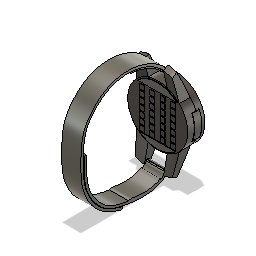
self-sus-wearable (Autodesk Fusion 360 design; units mm, degrees)
part number: Configuration 2
Autodesk Fusion 360 part; units mm, degrees
note: some values were not read from the file. Set by a fixed rule: which face or edge a step refers to.
(part 1 of 2)
sketch "Sketch1" plane through (0, 0, 0) normal (0, 1, 0) x (1, 0, 0)
  line L0 (0, 0) -> (0, 36)
  line L1 (0, 36) -> (-13.5946, 42.3393)
  line L2 (-13.5946, 42.3393) -> (-13.5946, 41.2357)
  line L3 (-13.5946, 41.2357) -> (-13.5946, 31.2357)
  line L4 (-13.5946, 31.2357) -> (-17.5946, 31.2357)
  line L5 (-17.5946, 31.2357) -> (-17.5946, 0)
  line L6 (-17.5946, 0) -> (0, 0)
  line L7 (-62.5946, 50) -> (-62.5946, 0)
  dimension "d1" = 36
  dimension "d2" = 15
  dimension "d5" = 65
  dimension "d6" = 10
  dimension "d7" = 4
  dimension "d11" = 45
  dimension "d12" = 31.2357
  constraint coincident L0.start L6.end
  constraint vertical L0
  constraint vertical L3
  constraint perpendicular L3 L4
  constraint perpendicular L4 L5
  constraint perpendicular L0 L6
  constraint vertical L7
  measures "d1" distance of L0.start L0.end
  measures "d2" distance of L0.end L1.end
  measures "d5" angle of L0 L1
  measures "d6" distance of L2.end L3.end
  measures "d7" distance of L3.end L4.end
  measures "d11" distance of L5 L7
  measures "d12" distance of L4.end L5.end
sketch "Sketch2" plane through (0, 0, 0) normal (0, 1, 0) x (1, 0, 0)
  line L0 (-62.5946, 45) -> (-62.5946, 0)
  line L1 (-17.5946, 31.2357) -> (-17.5946, 0)
  line L2 (0, 36) -> (-13.5946, 42.3393)
  dimension "d8" = 45
  constraint vertical L0
  measures "d8" distance of L0 L1
revolve "Revolve1" add sketch "Sketch1" angle 360 about axis through (-62.5946, 0, -45) along (0, 0, 1) makes body 1
sketch "Sketch3" plane through (0, 0, 0) normal (1, 0, 0) x (0, 0, -1)
  line L0 (20, 0) -> (7.7499, 0)
  line L1 (20, 0) -> (21.7425, 0)
  constraint horizontal L0
sketch "Sketch4" plane through (0, 0, 0) normal (0, 1, 0) x (1, 0, 0)
  line L0 (0.0672, 22.9643) -> (40, 1.7316)
  line L1 (40, 1.7316) -> (34.8066, -8.0357)
  line L2 (34.8066, -8.0357) -> (0, 0)
  line L3 (1.75, 0) -> (22.5, 0)
  line L4 (0, 20) -> (0, 7.7499)
  line L5 (0.0672, 22.9643) -> (0, 0)
  dimension "d14" = 13
  dimension "d15" = 28
  dimension "d16" = 40
  dimension "d17" = 31
  constraint perpendicular L0 L1
  constraint coincident L2.end L5.end
  measures "d14" angle of L2 L3
  measures "d15" angle of L0 L3
  measures "d16" distance of L0.end L4
  measures "d17" vertical distance of L0.start L1.end
revolve "Revolve2" add sketch "Sketch4" angle 360 about axis through (-62.5946, 0, 0) along (0, 0, -1) bodies 1
sketch "Sketch5" plane through (0, 0, 0) normal (0, 1, 0) x (1, 0, 0)
  line L0 (-40, 0) -> (-50, 0)
  constraint horizontal L0
sketch "Sketch6" plane through (0, 0, 0) normal (0, 0, 1) x (1, 0, 0)
  line L0 (-42.5946, 123.9624) -> (-42.5946, -152.8292)
  line L1 (-82.5946, 130) -> (-82.5946, -169.4999)
  circle A0 centre (-62.5946, 0) radius 62.6618
  line L2 (-107.5946, 43.6062) -> (-95.8637, 127.0763)
  line L3 (-17.5946, 43.6062) -> (-27.9388, 117.2086)
  line L4 (-107.5946, -43.6062) -> (-96.3645, -123.5125)
  line L5 (-17.5946, -43.6062) -> (-28.9448, -124.3667)
  line L6 (-96.3645, -123.5125) -> (-210, -123.5125)
  line L7 (-82.5946, 130) -> (-42.5946, 123.9624)
  line L8 (-95.8637, 127.0763) -> (-218.3448, 126.9812)
  line L9 (-218.3448, 126.9812) -> (-210, -123.5125)
  line L10 (-28.9448, -124.3667) -> (55.3958, -121.557)
  line L11 (55.3958, -121.557) -> (116.8374, -119.5102)
  line L12 (116.8374, -119.5102) -> (108.9821, 116.2876)
  line L13 (108.9821, 116.2876) -> (-27.9388, 117.2086)
  line L14 (-82.5946, -169.4999) -> (-42.5946, -152.8292)
  dimension "d19" = 20
  dimension "d20" = 20
  dimension "d33" = 8
  dimension "d34" = 8
  dimension "d35" = 8
  dimension "d37" = 8
  dimension "d38" = 45
  dimension "d39" = 45
  dimension "d42" = 8
  constraint vertical L0
  constraint vertical L1
  constraint coincident A0 L2.start
  constraint coincident A0 L3.start
  constraint coincident A0 L4.start
  constraint coincident A0 L5.start
  constraint horizontal L6
  constraint perpendicular L9 L10
  constraint perpendicular L11 L12
  measures "d19" distance of L0 A0.centre
  measures "d20" distance of L1 A0.centre
  measures "d33" angle of L1 L2
  measures "d34" angle of L0 L3
  measures "d35" angle of L1 L4
  measures "d37" angle of L0 L5
  measures "d38" horizontal distance of A0.centre L4.start
  measures "d39" horizontal distance of A0.centre L5.start
  measures "d42" angle of L1 L2
ref_plane "WorkPlane1" through (-62.5946, 0, 0) normal (0, 0, -1) x (-1, 0, 0)
extrude "Extrude1" cut sketch "Sketch6" along normal mid plane 100 contours L0 L1 A0 L7 | L0 L1 A0 L14 | A0 L3 L5 L10 L11 L12 L13 | A0 L2 L4 L6 L8 L9 bodies 1
sketch "Sketch9" plane through (0, 0, 0) normal (0, 0, 1) x (1, 0, 0)
  circle A0 centre (-62.5946, 0) radius 62.5946
  circle A1 centre (-62.5946, 0) radius 45
  circle A2 centre (-62.5946, 0) radius 45
  constraint concentric A0 A2
extrude "Extrude2" add sketch "Sketch9" against normal blind 2 contours A1 A2 bodies 1
sketch "Sketch10" plane through (0, 0, -2) normal (0, 0, -1) x (-1, 0, 0)
  circle A0 centre (62.5946, 0) radius 45
  circle A1 centre (62.5946, 0) radius 1
  dimension "d47" = 2
  constraint concentric A0 A1
  measures "d47" diameter of A1
extrude "Extrude3" add sketch "Sketch10" along normal blind 12 contours A1 bodies 1
sketch "Sketch11" plane through (0, 0, -2) normal (0, 0, -1) x (-1, 0, 0)
  circle A0 centre (62.5946, 0) radius 1
  circle A1 centre (62.5946, 0) radius 45
  line L0 (64.4575, 0.7277) -> (89.9628, 31.5413)
  line L1 (61.2831, -1.51) -> (30.4695, 23.9953)
  line L2 (68.704, 13.6995) -> (81.6598, 29.3517)
  line L3 (53.1863, 11.6826) -> (37.6452, 24.5464)
  line L4 (89.9628, 31.5413) -> (88.9026, 30.2604)
  arc A2 (81.6598, 29.3517) -> (37.6452, 24.5464) centre (62.5946, 0) ccw
  arc A3 (68.704, 13.6995) -> (53.1863, 11.6826) centre (62.5946, 0) ccw
  arc A4 (88.9026, 30.2604) -> (30.4695, 23.9953) centre (62.5946, 0) ccw
  arc A5 (61.2831, -1.51) -> (64.4575, 0.7277) centre (62.5946, 0) ccw
  line L5 (107.5502, -2) -> (97.5502, -2)
  line L6 (97.5502, -2) -> (97.5502, 2)
  line L7 (97.5502, 2) -> (107.5502, 2)
  line L8 (107.5502, 2) -> (107.5502, -2)
  line L9 (62.5946, 0) -> (62.5946, -26.6223)
  line L10 (17.6391, -2) -> (27.6391, -2)
  line L11 (27.6391, -2) -> (27.6391, 2)
  line L12 (27.6391, 2) -> (17.6391, 2)
  line L13 (17.6391, 2) -> (17.6391, -2)
  dimension "d50" = 4
  dimension "d51" = 40
  dimension "d52" = 40
  dimension "d53" = 90
  dimension "d54" = 30
  dimension "d55" = 5
  dimension "d56" = 5
  dimension "d57" = 70
  dimension "d58" = 10
  dimension "d59" = 4
  constraint concentric A0 A5
  constraint concentric A4 A5
  constraint concentric A3 A5
  constraint parallel L0 L2
  constraint perpendicular L2 L3
  constraint concentric A2 A3
  constraint parallel L0 L4
  constraint horizontal L5
  constraint vertical L6
  constraint horizontal L7
  constraint vertical L8
  constraint coincident A1 L5.start
  constraint coincident A0.centre A1.centre
  constraint vertical L9
  constraint symmetric L5.start L9 L10.start
  constraint symmetric L5.end L9 L10.end
  constraint symmetric L6.end L9 L11.end
  constraint symmetric L7.end L9 L12.end
  measures "d50" diameter of A5
  measures "d51" distance of L0.start L0.end
  measures "d52" distance of L1.start L1.end
  measures "d53" angle of L0 L1
  measures "d54" diameter of A3
  measures "d55" distance of L1 L3
  measures "d56" distance of L0 L2
  measures "d57" diameter of A2
  measures "d58" distance of L5.start L5.end
  measures "d59" distance of L5.start L7.end
extrude "Extrude1'" add sketch "Sketch11" along normal blind 5 separate body contours L0 L1 A4 A5 makes body 2 in component "Component"
extrude "Extrude1''" add sketch "Sketch11" along normal blind 10 separate body contours L5 L6 L7 L8 | L10 L11 L12 L13 makes body 3 at (-100.8835, 2, -8.6667) makes body 4 at (-24.3057, 2, -5.3333) in component "Component'"
sketch "Sketch12" plane through (0, 0, -7) normal (0, 0, -1) x (-1, 0, 0)
  circle A0 centre (62.5946, 0) radius 1
  arc A1 (81.6598, 29.3517) -> (37.6452, 24.5464) centre (62.5946, 0) ccw
  line L0 (81.6598, 29.3517) -> (68.704, 13.6995)
  arc A2 (68.704, 13.6995) -> (53.1863, 11.6826) centre (62.5946, 0) ccw
  line L1 (53.1863, 11.6826) -> (37.6452, 24.5464)
  arc A3 (61.2831, -1.51) -> (64.4575, 0.7277) centre (62.5946, 0) ccw
  line L2 (64.4575, 0.7277) -> (88.9026, 30.2604)
  arc A4 (88.9026, 30.2604) -> (30.4695, 23.9953) centre (62.5946, 0) ccw
  line L3 (30.4695, 23.9953) -> (61.2831, -1.51)
  line L4 (62.5946, 0) -> (30.8678, 0)
  line L5 (64.4575, -0.7277) -> (88.9026, -30.2604)
  arc A5 (64.4575, -0.7277) -> (61.2831, 1.51) centre (62.5946, 0) ccw
  line L6 (30.4695, -23.9953) -> (61.2831, 1.51)
  arc A6 (53.1863, -11.6826) -> (68.704, -13.6995) centre (62.5946, 0) ccw
  line L7 (81.6598, -29.3517) -> (68.704, -13.6995)
  line L8 (53.1863, -11.6826) -> (37.6452, -24.5464)
  arc A7 (37.6452, -24.5464) -> (81.6598, -29.3517) centre (62.5946, 0) ccw
  arc A8 (30.4695, -23.9953) -> (88.9026, -30.2604) centre (62.5946, 0) ccw
  constraint coincident A0.centre A1.centre
  constraint horizontal L4
  constraint symmetric A1.start L4 L7.start
  constraint symmetric A1.end L4 L8.end
  constraint symmetric A1 L4 A7
  constraint symmetric L0.end L4 A6.end
  constraint symmetric A2.end L4 A6.start
  constraint symmetric A2 L4 A6
  constraint symmetric A3.start L4 A5.end
  constraint symmetric A3.end L4 L5.start
  constraint symmetric A3 L4 A5
  constraint symmetric L2.end L4 L5.end
  constraint symmetric A4.end L4 L6.start
  constraint symmetric A4 L4 A8
extrude "Extrude1'''" add sketch "Sketch12" along normal blind 5 separate body contours A3 L3 A5 L6 | A3 L3 L5 L6 A8 makes body 5 in component "Component''"
sketch "Sketch13" plane through (0, 0, -14) normal (0, 0, -1) x (-1, 0, 0)
  circle A0 centre (62.5946, 0) radius 1
  circle A1 centre (62.5946, 0) radius 2.0145
  constraint concentric A0 A1
extrude "Extrude2'" add sketch "Sketch13" against normal up to surface (2 mm away) bodies 5 in component "Component''"
sketch "Sketch14" plane through (0, 0, -12) normal (0, 0, -1) x (-1, 0, 0)
  line L0 (17.6391, 2) -> (17.6391, -2)
  line L1 (17.6391, -2) -> (27.6391, -2)
  line L2 (27.6391, -2) -> (27.6391, 2)
  line L3 (27.6391, 2) -> (17.6391, 2)
  circle A0 centre (62.5636, 0.0374) radius 45.1126
extrude "Extrude1''''" add sketch "Sketch14" along normal blind 2 separate body contours L0 L1 L2 L3 | A0 makes body 6 in component "Component'''"
sketch "Sketch15" plane through (0, 0, -14) normal (0, 0, -1) x (-1, 0, 0)
  circle A0 centre (62.5946, 0) radius 62.5946
  line L0 (75.3013, -25.2103) -> (75.3013, 25.2103)
  line L1 (75.3013, 25.2103) -> (5.3013, 25.2103)
  line L2 (5.3013, -25.2103) -> (75.3013, -25.2103)
  arc A1 (5.3013, 25.2103) -> (5.3013, -25.2103) centre (62.5946, 0) ccw
  arc A2 (5.3013, 25.2103) -> (5.3013, -25.2103) centre (62.5946, 0) ccw
  dimension "d79" = 70
  constraint coincident A0 L1.end
  constraint coincident A0 L2.start
  constraint perpendicular L0 L2
  constraint concentric A0 A1
  constraint coincident origin A1
  constraint concentric A0 A2
  measures "d79" distance of L1.end L0.end
extrude "Extrude1'''''" add sketch "Sketch15" along normal blind 15 separate body contours A0 L0 L1 L2 A1 A2 makes body 7 in component "Component''''"
ref_plane "WorkPlane3" through (-17.5946, 0, -30.7135) normal (-1, 0, 0) x (0, 1, 0)
sketch "Sketch16" plane through (-17.5946, 0, 0) normal (-1, 0, 0) x (0, 0, 1)
  line L0 (-14, 25.2103) -> (-14, -25.2103)
  line L1 (-14, -25.2103) -> (-29, -25.2103)
  line L2 (-29, 25.2103) -> (-29, -25.2103)
  line L3 (-29, 25.2103) -> (-14, 25.2103)
extrude "Extrude4" cut sketch "Sketch16" against normal blind 30 bodies 1
sketch "Sketch17" plane through (0, 0, -14) normal (0, 0, -1) x (-1, 0, 0)
  circle A0 centre (62.5636, 0.0374) radius 45.1126
  line L0 (75.3432, 43.302) -> (75.3432, -43.2272)
  constraint coincident A0 L0.start
  constraint coincident A0 L0.end
  constraint vertical L0
extrude "Extrude1''''''" add sketch "Sketch17" along normal blind 10 separate body contours A0 L0 picked at (91.1131, 1.2012) makes body 8 in component "Component'''''"
sketch "Sketch18" plane through (0, 0, -31.2357) normal (0, 0, -1) x (-1, 0, 0)
  circle A0 centre (62.5946, 0) radius 45
  circle A1 centre (62.5946, 0) radius 49
  circle A2 centre (62.5946, 0) radius 49
extrude "Extrude1'''''''" add sketch "Sketch18" along normal blind 10 separate body contours A0 | A1 A2 makes body 9 in component "Component''''''"
sketch "Sketch19" plane through (-42.5946, 0, 0) normal (-1, 0, 0) x (0, 0, 1)
  spline S0 degree 2 poles (-22.9643, 59.3844) (-15.0842, 75.0225) (-1.7316, 100.6263) knots 0 0 0 4.638692 4.638692 4.638692 weights 1 1.032675 1
  line L0 (-22.9643, 59.3844) -> (0.0155, 59.3844)
  spline S1 degree 2 poles (8.0357, 95.3257) (3.094, 73.4548) (0.0155, 59.3844) knots 0 0 0 3.680754 3.680754 3.680754 weights 1 1.026272 1.000129
  spline S2 degree 2 poles (-1.7316, 100.6263) (3.2842, 97.9072) (8.0357, 95.3257) knots 0 0 0 1.111294 1.111294 1.111294 weights 1 1.000351 1
  circle A0 centre (0.03, 90.0112) radius 2.5
  line L1 (-2.0018, -2.0163) -> (7.3253, -2.0163)
  dimension "d93" = 5
  constraint horizontal L1
  measures "d93" diameter of A0
extrude "Extrude5" add sketch "Sketch19" along normal up to surface (40 mm away) contours A0 bodies 1
ref_plane "WorkPlane4" through (-39.4479, 0, -21.5) normal (0, 1, 0) x (1, 0, 0)
sketch "Sketch20" plane through (0, 0, 0) normal (1, 0, 0) x (0, 0, -1)
sketch "Sketch21" plane through (-82.5946, 0, 0) normal (1, 0, 0) x (0, 0, -1)
  circle A0 centre (-0.03, 90.0112) radius 2.5
  spline S0 degree 2 poles (1.7316, 100.6263) (15.0842, 75.0225) (22.9643, 59.3844) knots 0 0 0 4.638692 4.638692 4.638692 weights 1 1.032675 1
  spline S1 degree 2 poles (-8.0357, 95.3257) (-3.2842, 97.9072) (1.7316, 100.6263) knots 0 0 0 1.111294 1.111294 1.111294 weights 1 1.000351 1
  spline S2 degree 2 poles (-0.0155, 59.3844) (-3.094, 73.4548) (-8.0357, 95.3257) knots 0.009045 0.009045 0.009045 3.689799 3.689799 3.689799 weights 1.000129 1.026272 1
  line L0 (-0.0155, 59.3844) -> (22.9643, 59.3844)
  spline S3 degree 5 poles (-0.03, 90.0112) (-1.1775, 91.5817) (-3.4861, 94.6103) (-6.9902, 98.8157) (-11.7447, 103.7475) (-17.825, 108.7899) (-24.0418, 112.7267) (-30.3929, 115.597) (-36.8741, 117.4703) (-43.4784, 118.458) (-50.1921, 118.6922) (-56.9885, 118.2985) (-63.823, 117.3723) (-70.6262, 115.9477) (-77.3048, 113.9944) (-83.7529, 111.4513) (-89.8608, 108.2523) (-95.5249, 104.3541) (-100.6573, 99.7652) (-105.1919, 94.538) (-109.0908, 88.7576) (-112.3496, 82.5316) (-115.0058, 75.9807) (-117.1366, 69.2259) (-118.8402, 62.3703) (-120.2217, 55.4819) (-121.378, 48.578) (-122.3808, 41.6028) (-123.2748, 34.4519) (-124.0786, 27.0054) (-124.7843, 19.1583) (-125.3577, 10.8515) (-125.7382, 2.1043) (-125.8467, -7.0048) (-125.5941, -16.3577) (-124.8894, -25.8159) (-123.6477, -35.2395) (-121.7988, -44.5069) (-119.295, -53.5329) (-116.1063, -62.2615) (-112.2167, -70.6604) (-108.5391, -77.1033) (-105.4624, -81.7782) (-103.2697, -84.8249) (-102.138, -86.3308) knots 0 0 0 0 0 0 0.025 0.05 0.075 0.1 0.125 0.15 0.175 0.2 0.225 0.25 0.275 0.3 0.325 0.35 0.375 0.4 0.425 0.45 0.475 0.5 0.525 0.55 0.575 0.6 0.625 0.65 0.675 0.7 0.725 0.75 0.775 0.8 0.825 0.85 0.875 0.9 0.925 0.95 0.975 1 1 1 1 1 1
  spline S4 degree 5 poles (-0.03, -88.7812) (-0.131, -89.7768) (-0.4611, -91.6893) (-1.3406, -94.3212) (-3.2824, -97.3566) (-6.965, -100.3711) (-11.8136, -102.6418) (-17.6448, -104.2438) (-24.1432, -105.3074) (-30.9222, -105.9898) (-37.59, -106.4448) (-43.8164, -106.7917) (-49.3922, -107.0877) (-54.3102, -107.2902) (-58.7776, -107.2525) (-63.0946, -106.787) (-67.5661, -105.7115) (-72.3911, -103.9067) (-77.5872, -101.3554) (-83.048, -98.107) (-88.5838, -94.2512) (-93.9689, -89.8884) (-98.9836, -85.1033) (-103.4645, -79.9315) (-107.3087, -74.3724) (-110.4665, -68.4147) (-112.9385, -62.0574) (-114.7711, -55.3334) (-116.0525, -48.3294) (-116.9102, -41.2149) (-117.4903, -34.2046) (-117.9334, -27.5087) (-118.3511, -21.2887) (-118.8026, -15.6101) (-119.2715, -10.3958) (-119.6409, -5.3791) (-119.7526, -0.2294) (-119.4679, 5.3139) (-118.7236, 11.3211) (-117.6011, 17.5216) (-116.3584, 23.2381) (-115.5195, 26.7863) (-115.1006, 28.5643) (-114.9316, 29.3158) (-114.8746, 29.5831) knots 0 0 0 0 0 0 0.025 0.05 0.075 0.1 0.125 0.15 0.175 0.2 0.225 0.25 0.275 0.3 0.325 0.35 0.375 0.4 0.425 0.45 0.475 0.5 0.525 0.55 0.575 0.6 0.625 0.65 0.675 0.7 0.725 0.75 0.775 0.8 0.825 0.85 0.875 0.9 0.925 0.95 0.975 1 1 1 1 1 1
  line L1 (-116.3658, 22.5864) -> (-113.3834, 36.5799)
  line L2 (-2.0161, 88.4928) -> (1.8848, 91.6186)
  line L3 (1.8848, 91.6186) -> (0.0088, 93.9597)
  line L4 (0.0088, 93.9597) -> (-3.892, 90.8339)
  line L5 (-3.892, 90.8339) -> (-2.0161, 88.4928)
  line L6 (0, 0) -> (-17.413, 0)
  point P0 (-0.03, 90.0112)
  point P1 (-0.03, -88.7812)
  point P2 (-31.4782, 115.7247)
  point P3 (-60.8536, 117.7095)
  point P4 (-90.2291, 107.7854)
  point P5 (-110.8713, 85.1583)
  point P6 (-120.3985, 54.195)
  point P7 (-124.7651, 18.8651)
  point P8 (-123.5742, -34.7253)
  point P9 (-12.4238, -102.6064)
  point P10 (-47.3568, -106.9731)
  point P11 (-66.8081, -105.7822)
  point P12 (-94.9927, -88.7812)
  point P13 (-114.8746, -54.1766)
  point P14 (-118.8106, -15.671)
  point P15 (-118.8106, 10.1318)
  dimension "d96" = 3
  constraint coincident P0 A0.centre
  constraint coincident P1 S4.start
  constraint midpoint S4.end L1
  constraint perpendicular L2 L3
  constraint parallel L2 L4
  constraint parallel L3 L5
  constraint coincident A0 L2.end
  constraint coincident A0 L2.start
  constraint coincident L6.start origin
  constraint horizontal L6
  measures "d96" distance of L2 L4
extrude "Extrude6" add sketch "Sketch21" along normal up to surface (40 mm away) separate body contours A0 S3 L3 L4 | A0 S3 L4 L5 makes body 10
sketch "Sketch22" plane through (-82.5946, 0, 0) normal (1, 0, 0) x (0, 0, -1)
  circle A0 centre (-0.03, 90.0112) radius 2.5
  spline S0 degree 2 poles (1.7316, 100.6263) (15.0842, 75.0225) (22.9643, 59.3844) knots 0 0 0 4.638692 4.638692 4.638692 weights 1 1.032675 1
  spline S1 degree 2 poles (-8.0357, 95.3257) (-3.2842, 97.9072) (1.7316, 100.6263) knots 0 0 0 1.111294 1.111294 1.111294 weights 1 1.000351 1
  spline S2 degree 2 poles (-0.0155, 59.3844) (-3.094, 73.4548) (-8.0357, 95.3257) knots 0.009045 0.009045 0.009045 3.689799 3.689799 3.689799 weights 1.000129 1.026272 1
  line L0 (-0.0155, 59.3844) -> (22.9643, 59.3844)
  spline S3 degree 5 poles (-0.03, 90.0112) (-0.6767, 90.8889) (-2.0291, 92.6461) (-4.2351, 95.2872) (-7.5312, 98.8191) (-12.2518, 103.2421) (-17.5975, 107.645) (-23.6175, 111.9702) (-30.3859, 116.125) (-37.9718, 119.9894) (-46.4144, 123.4222) (-55.6978, 126.2675) (-65.7213, 128.36) (-76.2858, 129.5344) (-87.1316, 129.644) (-97.9676, 128.5791) (-108.5038, 126.2847) (-118.4815, 122.7787) (-127.7057, 118.171) (-136.0755, 112.6811) (-143.5614, 106.5855) (-150.1839, 100.1693) (-155.9914, 93.673) (-161.0404, 87.248) (-165.3699, 80.892) (-168.9954, 74.4501) (-171.9292, 67.7029) (-174.1945, 60.4338) (-175.8411, 52.5017) (-176.9632, 43.9206) (-177.6787, 34.8214) (-178.1037, 25.3995) (-178.3275, 15.8656) (-178.3905, 6.3998) (-178.2526, -2.907) (-177.7966, -12.0607) (-176.8674, -21.1141) (-175.3023, -30.1329) (-172.9649, -39.155) (-169.7771, -48.1533) (-165.7531, -56.9942) (-160.9787, -65.4778) (-155.5873, -73.3798) (-149.737, -80.4943) (-143.5891, -86.6726) (-137.2821, -91.8733) (-130.9187, -96.1758) (-124.5741, -99.7279) (-118.2996, -102.7059) (-112.1281, -105.2732) (-106.0791, -107.5325) (-101.3454, -109.1339) (-97.8559, -110.227) (-95.5565, -110.9077) (-94.4136, -111.236) knots 0 0 0 0 0 0 0.02 0.04 0.06 0.08 0.1 0.12 0.14 0.16 0.18 0.2 0.22 0.24 0.26 0.28 0.3 0.32 0.34 0.36 0.38 0.4 0.42 0.44 0.46 0.48 0.5 0.52 0.54 0.56 0.58 0.6 0.62 0.64 0.66 0.68 0.7 0.72 0.74 0.76 0.78 0.8 0.82 0.84 0.86 0.88 0.9 0.92 0.94 0.96 0.98 1 1 1 1 1 1
  spline S4 degree 5 poles (-0.03, -91.3957) (-0.4427, -92.2245) (-1.3184, -93.8318) (-2.783, -96.0917) (-5.0379, -98.8028) (-8.3673, -101.6874) (-12.2252, -104.0682) (-16.6482, -105.9476) (-21.6833, -107.3324) (-27.3471, -108.2396) (-33.5931, -108.7011) (-40.2762, -108.769) (-47.116, -108.5207) (-53.777, -108.0445) (-59.9469, -107.424) (-65.4194, -106.7233) (-70.1679, -105.9726) (-74.4427, -105.151) (-78.6547, -104.2014) (-83.2314, -103.0518) (-88.4766, -101.6336) (-94.4426, -99.9006) (-101.0054, -97.8224) (-107.9238, -95.3805) (-114.9065, -92.5638) (-121.6712, -89.364) (-128.0184, -85.7707) (-133.8388, -81.7703) (-139.086, -77.348) (-143.7603, -72.4877) (-147.8878, -67.1741) (-151.502, -61.3927) (-154.6244, -55.1316) (-157.2694, -48.3868) (-159.448, -41.1686) (-161.1727, -33.5072) (-162.4607, -25.4586) (-163.3393, -17.1113) (-163.8492, -8.5912) (-164.0403, -0.0497) (-163.9677, 8.3492) (-163.6872, 16.44) (-163.2512, 24.0691) (-162.7047, 31.1056) (-162.0804, 37.4561) (-161.3975, 43.0676) (-160.8121, 46.9452) (-160.3526, 49.5061) (-160.0371, 51.0592) (-159.8771, 51.7972) knots 0 0 0 0 0 0 0.022222 0.044444 0.066667 0.088889 0.111111 0.133333 0.155556 0.177778 0.2 0.222222 0.244444 0.266667 0.288889 0.311111 0.333333 0.355556 0.377778 0.4 0.422222 0.444444 0.466667 0.488889 0.511111 0.533333 0.555556 0.577778 0.6 0.622222 0.644444 0.666667 0.688889 0.711111 0.733333 0.755556 0.777778 0.8 0.822222 0.844444 0.866667 0.888889 0.911111 0.933333 0.955556 0.977778 1 1 1 1 1 1
  point P0 (-16.3029, 106.4839)
  point P1 (-53.4523, 125.4306)
  point P2 (-118.0426, 122.6097)
  point P3 (-158.7822, 90.0112)
  point P4 (-174.2633, 59.3844)
  point P5 (-178.3373, 10.983)
  point P6 (-172.6337, -39.5342)
  point P7 (-145.7455, -84.3478)
  point P8 (-117.2278, -103.0881)
  point P9 (-10.8171, -103.0881)
  point P10 (-33.7634, -108.6055)
  point P11 (-65.9381, -106.6101)
  point P12 (-83.0005, -103.0881)
  point P13 (-117.2278, -91.3957)
  point P14 (-147.6745, -67.1785)
  point P15 (-162.3177, -25.6895)
  point P16 (-162.9278, 28.0021)
sweep "Sweep1" add 2 faces at (-55.928, 92.9582, 1.241) (-69.2613, 91.9162, 2.5413) path "Sketch22" along S3 separate body on bodies 10 makes body 11 in component "Component'''''''"
mirror "Mirror1" about plane through (0, 0, 0) normal (0, 1, 0) of "Extrude5", "Extrude6" makes body 12
sketch "Sketch23" plane through (-82.5946, 0, 0) normal (1, 0, 0) x (0, 0, -1)
  circle A0 centre (-0.03, -90.0112) radius 2.5
  spline S0 degree 2 poles (-8.0357, -95.3257) (-3.094, -73.4548) (-0.0155, -59.3844) knots 0 0 0 3.680754 3.680754 3.680754 weights 1 1.026272 1.000129
  spline S1 degree 2 poles (1.7316, -100.6263) (-3.2842, -97.9072) (-8.0357, -95.3257) knots 0 0 0 1.111294 1.111294 1.111294 weights 1 1.000351 1
  spline S2 degree 2 poles (22.9643, -59.3844) (15.0842, -75.0225) (1.7316, -100.6263) knots 0 0 0 4.638692 4.638692 4.638692 weights 1 1.032675 1
  line L0 (22.9643, -59.3844) -> (-0.0155, -59.3844)
  circle A1 centre (-0.03, -90.0112) radius 2.5
  constraint concentric A0 A1
sketch "Sketch24" plane through (-82.5946, 0, 0) normal (1, 0, 0) x (0, 0, -1)
  spline S0 degree 5 poles (-0.0346, -90.0344) (-0.294, -90.7063) (-0.901, -92.0352) (-2.0767, -93.9835) (-4.1751, -96.4911) (-7.6849, -99.4634) (-12.0819, -102.2403) (-17.3639, -104.7526) (-23.5174, -106.9066) (-30.5067, -108.6047) (-38.2624, -109.7638) (-46.6725, -110.3329) (-55.5666, -110.3164) (-64.7224, -109.7746) (-73.8945, -108.7985) (-82.839, -107.4918) (-91.3379, -105.9497) (-99.2258, -104.2387) (-106.4121, -102.3784) (-112.9147, -100.3149) (-118.839, -97.9385) (-124.3344, -95.1202) (-129.5572, -91.7437) (-134.6343, -87.7349) (-139.6172, -83.1027) (-144.4814, -77.9333) (-149.1543, -72.3547) (-153.5359, -66.5101) (-157.5211, -60.5277) (-161.0229, -54.4911) (-163.992, -48.414) (-166.4116, -42.2699) (-168.2942, -36.0158) (-169.6774, -29.6193) (-170.6203, -23.0825) (-171.2008, -16.4706) (-171.5065, -9.8939) (-171.6264, -3.4844) (-171.6421, 2.6254) (-171.6192, 8.3231) (-171.5978, 13.5414) (-171.5976, 17.3068) (-171.61, 19.8962) (-171.6237, 21.5184) (-171.632, 22.3034) knots 0 0 0 0 0 0 0.025 0.05 0.075 0.1 0.125 0.15 0.175 0.2 0.225 0.25 0.275 0.3 0.325 0.35 0.375 0.4 0.425 0.45 0.475 0.5 0.525 0.55 0.575 0.6 0.625 0.65 0.675 0.7 0.725 0.75 0.775 0.8 0.825 0.85 0.875 0.9 0.925 0.95 0.975 1 1 1 1 1 1
  point P0 (-9.0728, -100.2262)
  point P1 (-42.7562, -109.9895)
  point P2 (-101.3361, -103.6433)
  point P3 (-131.6024, -90.0344)
  point P4 (-156.9871, -61.1729)
  point P5 (-169.6794, -28.954)
  point P6 (-171.632, 3.265)
sweep "Sweep1'" add 2 faces at (-55.928, -92.9582, 1.241) (-69.2613, -91.9162, 2.5413) path "Sketch24" along S0 separate body on bodies 12 makes body 13 in component "Component''''''''"
sketch "Sketch25" plane through (0, 0, 0) normal (0, 0, 1) x (1, 0, 0)
  circle A0 centre (-62.5946, 0) radius 62.5946
  line L0 (-25.0235, -45.0228) -> (-34.9304, -45.0228)
  line L1 (-34.9304, -45.0228) -> (-34.9304, -34.8918)
  line L2 (-34.9304, -34.8918) -> (-25.0235, -34.8918)
  line L3 (-25.0235, -34.8918) -> (-25.0235, -45.0228)
  line L4 (-41.2735, -34.8918) -> (-41.2735, -45.0228)
  line L5 (-41.2735, -45.0228) -> (-51.1804, -45.0228)
  line L6 (-51.1804, -45.0228) -> (-51.1804, -34.8918)
  line L7 (-51.1804, -34.8918) -> (-41.2735, -34.8918)
  line L8 (-57.5235, -34.8918) -> (-57.5235, -45.0228)
  line L9 (-57.5235, -45.0228) -> (-67.4304, -45.0228)
  line L10 (-67.4304, -45.0228) -> (-67.4304, -34.8918)
  line L11 (-67.4304, -34.8918) -> (-57.5235, -34.8918)
  line L12 (-73.7735, -34.8918) -> (-73.7735, -45.0228)
  line L13 (-73.7735, -45.0228) -> (-83.6804, -45.0228)
  line L14 (-83.6804, -45.0228) -> (-83.6804, -34.8918)
  line L15 (-83.6804, -34.8918) -> (-73.7735, -34.8918)
  line L16 (-90.0235, -34.8918) -> (-90.0235, -45.0228)
  line L17 (-90.0235, -45.0228) -> (-99.9304, -45.0228)
  line L18 (-99.9304, -45.0228) -> (-99.9304, -34.8918)
  line L19 (-99.9304, -34.8918) -> (-90.0235, -34.8918)
  line L20 (-25.0235, -21.5585) -> (-25.0235, -31.6895)
  line L21 (-25.0235, -31.6895) -> (-34.9304, -31.6895)
  line L22 (-34.9304, -31.6895) -> (-34.9304, -21.5585)
  line L23 (-34.9304, -21.5585) -> (-25.0235, -21.5585)
  line L24 (-41.2735, -21.5585) -> (-41.2735, -31.6895)
  line L25 (-41.2735, -31.6895) -> (-51.1804, -31.6895)
  line L26 (-51.1804, -31.6895) -> (-51.1804, -21.5585)
  line L27 (-51.1804, -21.5585) -> (-41.2735, -21.5585)
  line L28 (-57.5235, -21.5585) -> (-57.5235, -31.6895)
  line L29 (-57.5235, -31.6895) -> (-67.4304, -31.6895)
  line L30 (-67.4304, -31.6895) -> (-67.4304, -21.5585)
  line L31 (-67.4304, -21.5585) -> (-57.5235, -21.5585)
  line L32 (-73.7735, -21.5585) -> (-73.7735, -31.6895)
  line L33 (-73.7735, -31.6895) -> (-83.6804, -31.6895)
  line L34 (-83.6804, -31.6895) -> (-83.6804, -21.5585)
  line L35 (-83.6804, -21.5585) -> (-73.7735, -21.5585)
  line L36 (-90.0235, -21.5585) -> (-90.0235, -31.6895)
  line L37 (-90.0235, -31.6895) -> (-99.9304, -31.6895)
  line L38 (-99.9304, -31.6895) -> (-99.9304, -21.5585)
  line L39 (-99.9304, -21.5585) -> (-90.0235, -21.5585)
  line L40 (-25.0235, -8.2252) -> (-25.0235, -18.3561)
  line L41 (-25.0235, -18.3561) -> (-34.9304, -18.3561)
  line L42 (-34.9304, -18.3561) -> (-34.9304, -8.2252)
  line L43 (-34.9304, -8.2252) -> (-25.0235, -8.2252)
  line L44 (-41.2735, -8.2252) -> (-41.2735, -18.3561)
  line L45 (-41.2735, -18.3561) -> (-51.1804, -18.3561)
  line L46 (-51.1804, -18.3561) -> (-51.1804, -8.2252)
  line L47 (-51.1804, -8.2252) -> (-41.2735, -8.2252)
  line L48 (-57.5235, -8.2252) -> (-57.5235, -18.3561)
  line L49 (-57.5235, -18.3561) -> (-67.4304, -18.3561)
  line L50 (-67.4304, -18.3561) -> (-67.4304, -8.2252)
  line L51 (-67.4304, -8.2252) -> (-57.5235, -8.2252)
  line L52 (-73.7735, -8.2252) -> (-73.7735, -18.3561)
  line L53 (-73.7735, -18.3561) -> (-83.6804, -18.3561)
  line L54 (-83.6804, -18.3561) -> (-83.6804, -8.2252)
  line L55 (-83.6804, -8.2252) -> (-73.7735, -8.2252)
  line L56 (-90.0235, -8.2252) -> (-90.0235, -18.3561)
  line L57 (-90.0235, -18.3561) -> (-99.9304, -18.3561)
  line L58 (-99.9304, -18.3561) -> (-99.9304, -8.2252)
  line L59 (-99.9304, -8.2252) -> (-90.0235, -8.2252)
  line L60 (-25.0235, 5.1082) -> (-25.0235, -5.0228)
  line L61 (-25.0235, -5.0228) -> (-34.9304, -5.0228)
  line L62 (-34.9304, -5.0228) -> (-34.9304, 5.1082)
  line L63 (-34.9304, 5.1082) -> (-25.0235, 5.1082)
  line L64 (-41.2735, 5.1082) -> (-41.2735, -5.0228)
  line L65 (-41.2735, -5.0228) -> (-51.1804, -5.0228)
  line L66 (-51.1804, -5.0228) -> (-51.1804, 5.1082)
  line L67 (-51.1804, 5.1082) -> (-41.2735, 5.1082)
  line L68 (-57.5235, 5.1082) -> (-57.5235, -5.0228)
  line L69 (-57.5235, -5.0228) -> (-67.4304, -5.0228)
  line L70 (-67.4304, -5.0228) -> (-67.4304, 5.1082)
  line L71 (-67.4304, 5.1082) -> (-57.5235, 5.1082)
  line L72 (-73.7735, 5.1082) -> (-73.7735, -5.0228)
  line L73 (-73.7735, -5.0228) -> (-83.6804, -5.0228)
  line L74 (-83.6804, -5.0228) -> (-83.6804, 5.1082)
  line L75 (-83.6804, 5.1082) -> (-73.7735, 5.1082)
  line L76 (-90.0235, 5.1082) -> (-90.0235, -5.0228)
  line L77 (-90.0235, -5.0228) -> (-99.9304, -5.0228)
  line L78 (-99.9304, -5.0228) -> (-99.9304, 5.1082)
  line L79 (-99.9304, 5.1082) -> (-90.0235, 5.1082)
  line L80 (-25.0235, 18.4415) -> (-25.0235, 8.3105)
  line L81 (-25.0235, 8.3105) -> (-34.9304, 8.3105)
  line L82 (-34.9304, 8.3105) -> (-34.9304, 18.4415)
  line L83 (-34.9304, 18.4415) -> (-25.0235, 18.4415)
  line L84 (-41.2735, 18.4415) -> (-41.2735, 8.3105)
  line L85 (-41.2735, 8.3105) -> (-51.1804, 8.3105)
  line L86 (-51.1804, 8.3105) -> (-51.1804, 18.4415)
  line L87 (-51.1804, 18.4415) -> (-41.2735, 18.4415)
  line L88 (-57.5235, 18.4415) -> (-57.5235, 8.3105)
  line L89 (-57.5235, 8.3105) -> (-67.4304, 8.3105)
  line L90 (-67.4304, 8.3105) -> (-67.4304, 18.4415)
  line L91 (-67.4304, 18.4415) -> (-57.5235, 18.4415)
  line L92 (-73.7735, 18.4415) -> (-73.7735, 8.3105)
  line L93 (-73.7735, 8.3105) -> (-83.6804, 8.3105)
  line L94 (-83.6804, 8.3105) -> (-83.6804, 18.4415)
  line L95 (-83.6804, 18.4415) -> (-73.7735, 18.4415)
  line L96 (-90.0235, 18.4415) -> (-90.0235, 8.3105)
  line L97 (-90.0235, 8.3105) -> (-99.9304, 8.3105)
  line L98 (-99.9304, 8.3105) -> (-99.9304, 18.4415)
  line L99 (-99.9304, 18.4415) -> (-90.0235, 18.4415)
  line L100 (-25.0235, 31.7748) -> (-25.0235, 21.6439)
  line L101 (-25.0235, 21.6439) -> (-34.9304, 21.6439)
  line L102 (-34.9304, 21.6439) -> (-34.9304, 31.7748)
  line L103 (-34.9304, 31.7748) -> (-25.0235, 31.7748)
  line L104 (-41.2735, 31.7748) -> (-41.2735, 21.6439)
  line L105 (-41.2735, 21.6439) -> (-51.1804, 21.6439)
  line L106 (-51.1804, 21.6439) -> (-51.1804, 31.7748)
  line L107 (-51.1804, 31.7748) -> (-41.2735, 31.7748)
  line L108 (-57.5235, 31.7748) -> (-57.5235, 21.6439)
  line L109 (-57.5235, 21.6439) -> (-67.4304, 21.6439)
  line L110 (-67.4304, 21.6439) -> (-67.4304, 31.7748)
  line L111 (-67.4304, 31.7748) -> (-57.5235, 31.7748)
  line L112 (-73.7735, 31.7748) -> (-73.7735, 21.6439)
  line L113 (-73.7735, 21.6439) -> (-83.6804, 21.6439)
  line L114 (-83.6804, 21.6439) -> (-83.6804, 31.7748)
  line L115 (-83.6804, 31.7748) -> (-73.7735, 31.7748)
  line L116 (-90.0235, 31.7748) -> (-90.0235, 21.6439)
  line L117 (-90.0235, 21.6439) -> (-99.9304, 21.6439)
  line L118 (-99.9304, 21.6439) -> (-99.9304, 31.7748)
  line L119 (-99.9304, 31.7748) -> (-90.0235, 31.7748)
  line L120 (-25.0235, 45.1082) -> (-25.0235, 34.9772)
  line L121 (-25.0235, 34.9772) -> (-34.9304, 34.9772)
  line L122 (-34.9304, 34.9772) -> (-34.9304, 45.1082)
  line L123 (-34.9304, 45.1082) -> (-25.0235, 45.1082)
  line L124 (-41.2735, 45.1082) -> (-41.2735, 34.9772)
  line L125 (-41.2735, 34.9772) -> (-51.1804, 34.9772)
  line L126 (-51.1804, 34.9772) -> (-51.1804, 45.1082)
  line L127 (-51.1804, 45.1082) -> (-41.2735, 45.1082)
  line L128 (-57.5235, 45.1082) -> (-57.5235, 34.9772)
  line L129 (-57.5235, 34.9772) -> (-67.4304, 34.9772)
  line L130 (-67.4304, 34.9772) -> (-67.4304, 45.1082)
  line L131 (-67.4304, 45.1082) -> (-57.5235, 45.1082)
  line L132 (-73.7735, 45.1082) -> (-73.7735, 34.9772)
  line L133 (-73.7735, 34.9772) -> (-83.6804, 34.9772)
  line L134 (-83.6804, 34.9772) -> (-83.6804, 45.1082)
  line L135 (-83.6804, 45.1082) -> (-73.7735, 45.1082)
  line L136 (-90.0235, 45.1082) -> (-90.0235, 34.9772)
  line L137 (-90.0235, 34.9772) -> (-99.9304, 34.9772)
  line L138 (-99.9304, 34.9772) -> (-99.9304, 45.1082)
  line L139 (-99.9304, 45.1082) -> (-90.0235, 45.1082)
  dimension "d115" = -65
  dimension "d116" = 80
  constraint horizontal L0
  constraint vertical L1
  constraint horizontal L2
  constraint vertical L3
extrude "Extrude7" add sketch "Sketch25" along normal blind 1 contours L0 L1 L2 L3 bodies 1 10 12
pattern_linear "R-Pattern1" count 4 spacing 21.6667 along (-1, 0, 0) count 7 spacing 12.5 along (0, 1, 0) of "Extrude7"
sketch "Sketch26" plane through (-42.5946, 0, 0) normal (1, 0, 0) x (0, 0, -1)
  spline S0 degree 3 poles (-3.892, -90.8339) (-5.2727, -93.1469) (-7.6138, -95.5218) (-10.9951, -97.7495) (-14.1546, -99.831) (-18.2042, -101.7722) (-23.0866, -103.328) (-27.6487, -104.7817) (-32.9459, -105.8898) (-38.8204, -106.5134) (-44.3094, -107.0961) (-50.3044, -107.2525) (-56.5013, -107.0266) (-62.2916, -106.8156) (-68.2472, -106.2789) (-74.0547, -105.5352) (-79.4812, -104.8403) (-84.7729, -103.9696) (-89.7237, -103.0064) (-94.3497, -102.1065) (-98.6748, -101.1284) (-102.6337, -100.0784) (-106.3328, -99.0972) (-109.7138, -98.0511) (-112.8385, -96.8809) (-118.6072, -94.7205) (-123.5357, -92.1148) (-128.3713, -88.5557) (-130.5014, -86.9879) (-132.6081, -85.2388) (-134.6992, -83.3175) (-138.5597, -79.7702) (-142.3719, -75.6314) (-145.9365, -71.2127) (-149.0389, -67.3668) (-151.9404, -63.3257) (-154.4896, -59.2695) (-156.7082, -55.7391) (-158.659, -52.1965) (-160.3112, -48.6416) (-163.1525, -42.5281) (-165.1011, -36.3457) (-166.3371, -29.851) (-167.2565, -25.0199) (-167.789, -20.014) (-168.0922, -15.014) (-168.3178, -11.2947) (-168.4192, -7.5884) (-168.4662, -4.0126) (-168.5353, 1.2429) (-168.4975, 6.1962) (-168.4824, 10.608) (-168.4677, 14.9134) (-168.4682, 18.7146) (-168.5001, 21.9817) knots 0.020993 0.020993 0.020993 0.020993 0.085226 0.085226 0.085226 0.145244 0.145244 0.145244 0.201324 0.201324 0.201324 0.253726 0.253726 0.253726 0.302689 0.302689 0.302689 0.348439 0.348439 0.348439 0.391188 0.391188 0.391188 0.431132 0.431132 0.431132 0.504878 0.504878 0.504878 0.537363 0.537363 0.537363 0.597338 0.597338 0.597338 0.649538 0.649538 0.649538 0.69497 0.69497 0.69497 0.773102 0.773102 0.773102 0.831221 0.831221 0.831221 0.874453 0.874453 0.874453 0.937993 0.937993 0.937993 1 1 1 1
  line L0 (-168.5001, 21.9817) -> (-173.4727, 22.4925)
  spline S1 degree 3 poles (0.0088, -93.9597) (-1.9523, -96.9971) (-4.8952, -99.7535) (-8.7766, -102.2289) (-12.4034, -104.5419) (-16.8698, -106.6059) (-22.1423, -108.2367) (-27.0689, -109.7605) (-32.704, -110.8914) (-38.8738, -111.5118) (-44.6388, -112.0916) (-50.8684, -112.223) (-57.2559, -111.968) (-63.2244, -111.7298) (-69.3219, -111.1624) (-75.2517, -110.3885) (-80.7924, -109.6654) (-86.1807, -108.7671) (-91.2321, -107.7721) (-95.9521, -106.8424) (-100.3743, -105.8314) (-104.4627, -104.7304) (-112.0106, -102.6979) (-118.4133, -100.354) (-124.2822, -97.0861) (-126.8674, -95.6466) (-129.3542, -94.0267) (-131.7886, -92.2039) (-134.0632, -90.5006) (-136.2927, -88.6206) (-138.4875, -86.5787) (-142.5395, -82.809) (-146.4823, -78.4844) (-150.1632, -73.8814) (-153.3669, -69.875) (-156.3595, -65.6721) (-159.0015, -61.4211) (-161.301, -57.7211) (-163.3339, -53.9818) (-165.0594, -50.204) (-166.5613, -46.916) (-167.8312, -43.595) (-168.8756, -40.2237) (-170.6718, -34.4259) (-171.7915, -28.4499) (-172.4557, -22.3993) (-173.4319, -13.5063) (-173.4766, -4.5083) (-173.4706, 3.3114) (-173.4676, 7.1736) (-173.4454, 10.7507) (-173.4405, 13.9866) (-173.4357, 17.1444) (-173.4451, 19.9814) (-173.4727, 22.4925) knots 0.020993 0.020993 0.020993 0.020993 0.085226 0.085226 0.085226 0.145244 0.145244 0.145244 0.201324 0.201324 0.201324 0.253726 0.253726 0.253726 0.302689 0.302689 0.302689 0.348439 0.348439 0.348439 0.391188 0.391188 0.391188 0.470112 0.470112 0.470112 0.504878 0.504878 0.504878 0.537363 0.537363 0.537363 0.597338 0.597338 0.597338 0.649538 0.649538 0.649538 0.69497 0.69497 0.69497 0.734513 0.734513 0.734513 0.802516 0.802516 0.802516 0.902464 0.902464 0.902464 0.951828 0.951828 0.951828 1 1 1 1
  spline S2 degree 3 poles (0.0088, -93.9597) (0.6498, -92.967) (1.1841, -91.9433) (1.6056, -90.8908) knots 0 0 0 0 0.020993 0.020993 0.020993 0.020993
  line L1 (1.6056, -90.8908) -> (-2.8254, -88.577)
  spline S3 degree 3 poles (-3.892, -90.8339) (-3.4408, -90.078) (-3.0888, -89.3269) (-2.8254, -88.577) knots 0 0 0 0 0.020993 0.020993 0.020993 0.020993
sketch "Sketch27" plane through (0, 0, 0) normal (0, 0, 1) x (1, 0, 0)
  line L0 (-90.0235, 40.1082) -> (-90.0235, 29.9772)
  line L1 (-90.0235, 29.9772) -> (-99.9304, 29.9772)
  line L2 (-99.9304, 29.9772) -> (-99.9304, 40.1082)
  line L3 (-99.9304, 40.1082) -> (-90.0235, 40.1082)
  line L4 (-68.3569, 40.1082) -> (-68.3569, 29.9772)
  line L5 (-68.3569, 29.9772) -> (-78.2637, 29.9772)
  line L6 (-78.2637, 29.9772) -> (-78.2637, 40.1082)
  line L7 (-78.2637, 40.1082) -> (-68.3569, 40.1082)
  line L8 (-46.6902, 40.1082) -> (-46.6902, 29.9772)
  line L9 (-46.6902, 29.9772) -> (-56.597, 29.9772)
  line L10 (-56.597, 29.9772) -> (-56.597, 40.1082)
  line L11 (-56.597, 40.1082) -> (-46.6902, 40.1082)
  line L12 (-25.0235, 40.1082) -> (-25.0235, 29.9772)
  line L13 (-25.0235, 29.9772) -> (-34.9304, 29.9772)
  line L14 (-34.9304, 29.9772) -> (-34.9304, 40.1082)
  line L15 (-34.9304, 40.1082) -> (-25.0235, 40.1082)
  line L16 (-90.0235, 27.6082) -> (-90.0235, 17.4772)
  line L17 (-90.0235, 17.4772) -> (-99.9304, 17.4772)
  line L18 (-99.9304, 17.4772) -> (-99.9304, 27.6082)
  line L19 (-99.9304, 27.6082) -> (-90.0235, 27.6082)
  line L20 (-68.3569, 27.6082) -> (-68.3569, 17.4772)
  line L21 (-68.3569, 17.4772) -> (-78.2637, 17.4772)
  line L22 (-78.2637, 17.4772) -> (-78.2637, 27.6082)
  line L23 (-78.2637, 27.6082) -> (-68.3569, 27.6082)
  line L24 (-46.6902, 27.6082) -> (-46.6902, 17.4772)
  line L25 (-46.6902, 17.4772) -> (-56.597, 17.4772)
  line L26 (-56.597, 17.4772) -> (-56.597, 27.6082)
  line L27 (-56.597, 27.6082) -> (-46.6902, 27.6082)
  line L28 (-25.0235, 27.6082) -> (-25.0235, 17.4772)
  line L29 (-25.0235, 17.4772) -> (-34.9304, 17.4772)
  line L30 (-34.9304, 17.4772) -> (-34.9304, 27.6082)
  line L31 (-34.9304, 27.6082) -> (-25.0235, 27.6082)
  line L32 (-90.0235, 15.1082) -> (-90.0235, 4.9772)
  line L33 (-90.0235, 4.9772) -> (-99.9304, 4.9772)
  line L34 (-99.9304, 4.9772) -> (-99.9304, 15.1082)
  line L35 (-99.9304, 15.1082) -> (-90.0235, 15.1082)
  line L36 (-68.3569, 15.1082) -> (-68.3569, 4.9772)
  line L37 (-68.3569, 4.9772) -> (-78.2637, 4.9772)
  line L38 (-78.2637, 4.9772) -> (-78.2637, 15.1082)
  line L39 (-78.2637, 15.1082) -> (-68.3569, 15.1082)
  line L40 (-46.6902, 15.1082) -> (-46.6902, 4.9772)
  line L41 (-46.6902, 4.9772) -> (-56.597, 4.9772)
  line L42 (-56.597, 4.9772) -> (-56.597, 15.1082)
  line L43 (-56.597, 15.1082) -> (-46.6902, 15.1082)
  line L44 (-25.0235, 15.1082) -> (-25.0235, 4.9772)
  line L45 (-25.0235, 4.9772) -> (-34.9304, 4.9772)
  line L46 (-34.9304, 4.9772) -> (-34.9304, 15.1082)
  line L47 (-34.9304, 15.1082) -> (-25.0235, 15.1082)
  line L48 (-90.0235, 2.6082) -> (-90.0235, -7.5228)
  line L49 (-90.0235, -7.5228) -> (-99.9304, -7.5228)
  line L50 (-99.9304, -7.5228) -> (-99.9304, 2.6082)
  line L51 (-99.9304, 2.6082) -> (-90.0235, 2.6082)
  line L52 (-68.3569, 2.6082) -> (-68.3569, -7.5228)
  line L53 (-68.3569, -7.5228) -> (-78.2637, -7.5228)
  line L54 (-78.2637, -7.5228) -> (-78.2637, 2.6082)
  line L55 (-78.2637, 2.6082) -> (-68.3569, 2.6082)
  line L56 (-46.6902, 2.6082) -> (-46.6902, -7.5228)
  line L57 (-46.6902, -7.5228) -> (-56.597, -7.5228)
  line L58 (-56.597, -7.5228) -> (-56.597, 2.6082)
  line L59 (-56.597, 2.6082) -> (-46.6902, 2.6082)
  line L60 (-25.0235, 2.6082) -> (-25.0235, -7.5228)
  line L61 (-25.0235, -7.5228) -> (-34.9304, -7.5228)
  line L62 (-34.9304, -7.5228) -> (-34.9304, 2.6082)
  line L63 (-34.9304, 2.6082) -> (-25.0235, 2.6082)
  line L64 (-90.0235, -9.8918) -> (-90.0235, -20.0228)
  line L65 (-90.0235, -20.0228) -> (-99.9304, -20.0228)
  line L66 (-99.9304, -20.0228) -> (-99.9304, -9.8918)
  line L67 (-99.9304, -9.8918) -> (-90.0235, -9.8918)
  line L68 (-68.3569, -9.8918) -> (-68.3569, -20.0228)
  line L69 (-68.3569, -20.0228) -> (-78.2637, -20.0228)
  line L70 (-78.2637, -20.0228) -> (-78.2637, -9.8918)
  line L71 (-78.2637, -9.8918) -> (-68.3569, -9.8918)
  line L72 (-46.6902, -9.8918) -> (-46.6902, -20.0228)
  line L73 (-46.6902, -20.0228) -> (-56.597, -20.0228)
  line L74 (-56.597, -20.0228) -> (-56.597, -9.8918)
  line L75 (-56.597, -9.8918) -> (-46.6902, -9.8918)
  line L76 (-25.0235, -9.8918) -> (-25.0235, -20.0228)
  line L77 (-25.0235, -20.0228) -> (-34.9304, -20.0228)
  line L78 (-34.9304, -20.0228) -> (-34.9304, -9.8918)
  line L79 (-34.9304, -9.8918) -> (-25.0235, -9.8918)
  line L80 (-90.0235, -22.3918) -> (-90.0235, -32.5228)
  line L81 (-90.0235, -32.5228) -> (-99.9304, -32.5228)
  line L82 (-99.9304, -32.5228) -> (-99.9304, -22.3918)
  line L83 (-99.9304, -22.3918) -> (-90.0235, -22.3918)
  line L84 (-68.3569, -22.3918) -> (-68.3569, -32.5228)
  line L85 (-68.3569, -32.5228) -> (-78.2637, -32.5228)
  line L86 (-78.2637, -32.5228) -> (-78.2637, -22.3918)
  line L87 (-78.2637, -22.3918) -> (-68.3569, -22.3918)
  line L88 (-46.6902, -22.3918) -> (-46.6902, -32.5228)
  line L89 (-46.6902, -32.5228) -> (-56.597, -32.5228)
  line L90 (-56.597, -32.5228) -> (-56.597, -22.3918)
  line L91 (-56.597, -22.3918) -> (-46.6902, -22.3918)
  line L92 (-25.0235, -22.3918) -> (-25.0235, -32.5228)
  line L93 (-25.0235, -32.5228) -> (-34.9304, -32.5228)
  line L94 (-34.9304, -32.5228) -> (-34.9304, -22.3918)
  line L95 (-34.9304, -22.3918) -> (-25.0235, -22.3918)
  line L96 (-90.0235, -34.8918) -> (-90.0235, -45.0228)
  line L97 (-90.0235, -45.0228) -> (-99.9304, -45.0228)
  line L98 (-99.9304, -45.0228) -> (-99.9304, -34.8918)
  line L99 (-99.9304, -34.8918) -> (-90.0235, -34.8918)
  line L100 (-68.3569, -34.8918) -> (-68.3569, -45.0228)
  line L101 (-68.3569, -45.0228) -> (-78.2637, -45.0228)
  line L102 (-78.2637, -45.0228) -> (-78.2637, -34.8918)
  line L103 (-78.2637, -34.8918) -> (-68.3569, -34.8918)
  line L104 (-46.6902, -34.8918) -> (-46.6902, -45.0228)
  line L105 (-46.6902, -45.0228) -> (-56.597, -45.0228)
  line L106 (-56.597, -45.0228) -> (-56.597, -34.8918)
  line L107 (-56.597, -34.8918) -> (-46.6902, -34.8918)
  line L108 (-25.0235, -34.8918) -> (-25.0235, -45.0228)
  line L109 (-25.0235, -45.0228) -> (-34.9304, -45.0228)
  line L110 (-34.9304, -45.0228) -> (-34.9304, -34.8918)
  line L111 (-34.9304, -34.8918) -> (-25.0235, -34.8918)
  circle A0 centre (-62.5946, 0) radius 62.5946
  circle A1 centre (-62.5946, 0) radius 60
  line L112 (-103.3966, 43.9909) -> (-21.7927, 43.9909)
  line L113 (-62.5946, 0) -> (-46.6902, 0)
  line L114 (-103.3966, -43.9909) -> (-21.7927, -43.9909)
  dimension "d128" = 120
  constraint concentric A0 A1
  constraint coincident A1 L112.start
  constraint coincident A1 L112.end
  constraint horizontal L112
  constraint coincident A0.centre A1.centre
  constraint coincident L56 L113.end
  constraint perpendicular L56 L113
  constraint symmetric L112.start L113 L114.start
  constraint symmetric L112.end L113 L114.end
  measures "d128" diameter of A1
extrude "Extrude1''''''''" add sketch "Sketch27" along normal blind 1.3 separate body contours L96 L97 L98 L100 L101 L102 L104 L105 L106 L108 L109 L110 A1 L114 | A1 L112 makes body 14 at (-62.5162, -50.0152, 0) makes body 15 at (-54.3642, 50.302, 0) in component "Component'''''''''"
sketch "Sketch28" plane through (0, 0, 1.3) normal (0, 0, 1) x (1, 0, 0)
  line L0 (-25.0235, -43.9909) -> (-25.0235, -45.0228)
  line L1 (-25.0235, -45.0228) -> (-34.9304, -45.0228)
  line L2 (-34.9304, -45.0228) -> (-34.9304, -43.9909)
  line L3 (-34.9304, -43.9909) -> (-46.6902, -43.9909)
  line L4 (-46.6902, -43.9909) -> (-46.6902, -45.0228)
  line L5 (-46.6902, -45.0228) -> (-56.597, -45.0228)
  line L6 (-56.597, -45.0228) -> (-56.597, -43.9909)
  line L7 (-56.597, -43.9909) -> (-68.3569, -43.9909)
  line L8 (-68.3569, -43.9909) -> (-68.3569, -45.0228)
  line L9 (-68.3569, -45.0228) -> (-78.2637, -45.0228)
  line L10 (-78.2637, -45.0228) -> (-78.2637, -43.9909)
  line L11 (-78.2637, -43.9909) -> (-90.0235, -43.9909)
  line L12 (-90.0235, -43.9909) -> (-90.0235, -45.0228)
  line L13 (-90.0235, -45.0228) -> (-99.9304, -45.0228)
  line L14 (-99.9304, -45.0228) -> (-99.9304, -43.9909)
  line L15 (-99.9304, -43.9909) -> (-103.3966, -43.9909)
  arc A0 (-103.3966, -43.9909) -> (-21.7927, -43.9909) centre (-62.5946, 0) ccw
  line L16 (-21.7927, -43.9909) -> (-25.0235, -43.9909)
  line L17 (-100.2267, -46.7314) -> (-24.2026, -46.1091)
  constraint coincident A0 L17.start
  constraint coincident A0 L17.end
extrude "Extrude2''" cut sketch "Sketch28" against normal up to surface (1.3 mm away) contours L0 L1 L2 L3 L4 L5 L6 L7 L8 L9 L10 L11 L12 L13 L14 L15 A0 L16 L17 bodies 14 in component "Component'''''''''"